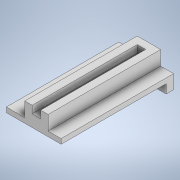
# Autodesk Inventor part: gyro_holder
Saved by Autodesk Inventor 2020 (Build 240168000, 168)
## iProperties
Created: 2019-06-18
Part Number: gyro_holder
Material: Generic
Document SubType Name: Modeling
Designer: erwin
Density: 1 g/cm^3
Appearance: Default
Author: erwin
Autodesk Inventor part; units mm, degrees
ref_plane "YZ Plane" through (0, 0, 0) normal (1, 0, 0) x (0, 1, 0)
ref_plane "XZ Plane" through (0, 0, 0) normal (0, 1, 0) x (-1, 0, 0)
ref_plane "XY Plane" through (0, 0, 0) normal (0, 0, 1) x (1, 0, 0)
sketch "Sketch1" plane through (0, 0, 0) normal (0, 1, 0) x (-1, 0, 0)
  line L0 (0.85, 10.55) -> (-0.85, 10.55)
  line L1 (-0.85, 10.55) -> (-0.85, -10.55)
  line L2 (-0.85, -10.55) -> (0.85, -10.55)
  line L3 (0.85, -10.55) -> (0.85, 10.55)
  line L4 (0.85, 10.55) -> (-0.85, -10.55) construction
  line L5 (-0.85, 10.55) -> (0.85, -10.55) construction
  line L6 (2.35, 12.05) -> (-2.35, 12.05)
  line L7 (-2.35, 12.05) -> (-2.35, -12.05)
  line L8 (-2.35, -12.05) -> (2.35, -12.05)
  line L9 (2.35, -12.05) -> (2.35, 12.05)
  point P0 (0, 0)
  dimension "d0" = 1.7
  dimension "d1" = 21.1
  dimension "d2" = 1.5
  constraints: 20 end point, 4 parallel, 2 midpoint, 2 perpendicular, 1 horizontal, 3 other
  measures "d0" distance of L2.end L1.end
  measures "d1" distance of L1.end L0.end
  measures "d2" distance between parallel lines of L3 L9
extrude "Extrusion1" add sketch "Sketch1" along normal blind 1.5
sketch "Sketch2" plane through (0, 0, 0) normal (0, -1, 0) x (1, 0, 0)
  line L0 (4.95, 12.05) -> (-6.05, 12.05)
  line L1 (-6.05, 12.05) -> (-6.05, -12.05)
  line L2 (-6.05, -12.05) -> (4.95, -12.05)
  line L3 (4.95, -12.05) -> (4.95, 12.05)
  line L4 (-2.35, 12.05) -> (2.35, 12.05) projected
  line L5 (-2.35, -12.05) -> (-2.35, 12.05) projected
  dimension "d5" = 11
  dimension "d6" = 3.7
  constraints: 8 end point, 2 parallel, 1 collinear, 1 horizontal, 1 perpendicular
  measures "d5" distance of L2.end L1.end
  measures "d6" distance between parallel lines of L5 L1
extrude "Extrusion2" add sketch "Sketch2" along normal blind 2.4
sketch "Sketch3" plane through (0, 0, 0) normal (0, 1, 0) x (1, 0, 0)
  line L0 (-2.35, 12.05) -> (-2.35, -12.05) projected
  line L1 (-6.05, 12.05) -> (-2.35, 12.05) projected
  line L2 (-6.05, -12.05) -> (-6.05, 12.05) projected
  line L3 (-2.35, -12.05) -> (-6.05, -12.05) projected
  line L4 (2.35, -12.05) -> (2.35, 12.05) projected
  line L5 (4.95, -12.05) -> (2.35, -12.05) projected
  line L6 (4.95, 12.05) -> (4.95, -12.05) projected
  line L7 (2.35, 12.05) -> (4.95, 12.05) projected
  point P0 (0, 0)
extrude "Extrusion3" cut sketch "Sketch3" against normal blind 1.4
move faces "Move1" translate (0, 0, -1.5) faces at (0.7833, 0.5333, 12.05)
sketch "Sketch4" plane through (0, -2.4, 0) normal (0, -1, 0) x (1, 0, 0)
  line L0 (-0.85, -10.55) -> (0.85, -10.55) projected
  line L1 (-6.05, 10.55) -> (-6.05, -12.05) projected
  line L2 (2.35, -12.05) -> (4.95, -12.05) projected
  line L3 (-6.05, -10.55) -> (4.95, -10.55)
  line L4 (4.95, -10.55) -> (4.95, -12.05)
  line L5 (4.95, -12.05) -> (-6.05, -12.05)
  line L6 (-6.05, -12.05) -> (-6.05, -10.55)
  point P0 (0, 0)
  constraints: 8 end point, 2 parallel, 1 horizontal, 1 perpendicular, 1 point on line
extrude "Extrusion4" add sketch "Sketch4" along normal blind 1.8
body "Solid1"
